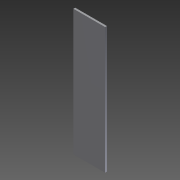
# Autodesk Inventor part: longeron
Saved by Autodesk Inventor 2011 (Build 150239000, 239)
## iProperties
Created: 2011-01-27
Part Number: longeron
Document SubType Name: Modeling
Designer: Physics Student
Density: 1 g/cm^3
Author: Physics Student
Autodesk Inventor part; units mm, degrees
ref_plane "YZ Plane" through (0, 0, 0) normal (1, 0, 0) x (0, 1, 0)
ref_plane "XZ Plane" through (0, 0, 0) normal (0, 1, 0) x (-1, 0, 0)
ref_plane "XY Plane" through (0, 0, 0) normal (0, 0, 1) x (1, 0, 0)
sketch "Sketch1" plane through (0, 0, 0) normal (0, 0, 1) x (1, 0, 0)
  line L0 (-40, 2.286) -> (40, 2.286)
  line L1 (40, 2.286) -> (40, -2.286)
  line L2 (40, -2.286) -> (-40, -2.286)
  line L3 (-40, -2.286) -> (-40, 2.286)
  line L4 (0, -14.5337) -> (0, 22.9692)
  line L5 (-9.7607, 0) -> (47.5072, 0)
  point P0 (0, 0)
  dimension "d0" = 80
  dimension "d1" = 0
  dimension "d2" = 4.572
  dimension "d5" = 0
  constraints: 12 end point, 3 parallel, 2 perpendicular, 1 horizontal, 2 other
  measures "d0" distance of L1.end L2.end
  measures "d1" distance from line of point (0, 0) L5
  measures "d2" distance between parallel lines of L2 L0
  measures "d5" distance from line of point (0, 0) L4
extrude "Extrusion1" add sketch "Sketch1" along normal blind 317.5
body "Solid1"
